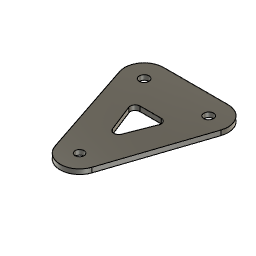
X Axis Support - Inside Support V2 (Autodesk Fusion 360 design; units mm, degrees)
Autodesk Fusion 360 part; units mm, degrees
sketch "Sketch1" plane through (0, 0, 0) normal (0, 0, 1) x (1, 0, 0) in component "X Axis Support - Inside Support V2"
  line L0 (0, 0) -> (64, 0)
  line L1 (64, 0) -> (64, 84)
  line L2 (64, 84) -> (0, 84)
  line L3 (0, 84) -> (0, 0)
  dimension "d1" = 64
  dimension "d2" = 84
  constraint horizontal L0
  constraint vertical L1
  constraint horizontal L2
  constraint vertical L3
  constraint coincident L0.start L3.end
  measures "d1" distance of L0.start L0.end
  measures "d2" distance of L0.start L2.end
extrude "Extrude1" add sketch "Sketch1" along normal blind 3 in component "X Axis Support - Inside Support V2"
sketch "Sketch2" plane through (0, 0, 3) normal (0, 0, 1) x (-1, 0, 0) in component "X Axis Support - Inside Support V2"
  line L0 (0, -84) -> (0, 0)
  line L1 (0, 0) -> (-64, 0)
  line L2 (-64, 0) -> (-64, -84)
  line L3 (-64, -84) -> (0, -84)
  line L4 (-12, -84) -> (-12, 0) construction
  line L5 (-52, -84) -> (-52, 0) construction
  line L6 (0, -12) -> (-64, -12) construction
  line L7 (0, -72) -> (-64, -72) construction
  circle A0 centre (-12, -72) radius 12
  circle A1 centre (-52, -72) radius 12
  circle A2 centre (-12, -72) radius 3
  circle A3 centre (-52, -72) radius 3
  line L8 (0, -72) -> (0, 0)
  line L9 (0, 0) -> (-32, 0)
  line L10 (-32, 0) -> (-64, 0)
  line L11 (-64, 0) -> (-64, -72)
  circle A4 centre (-32, -12) radius 12
  circle A5 centre (-32, -12) radius 2.75
  line L12 (0, -26) -> (-64, -26) construction
  line L13 (-12, 0) -> (0, -26)
  line L14 (-52, 0) -> (-64, -26)
  line L15 (0, -85) -> (-64, -85) construction
  line L16 (-32, -85) -> (-32, 0) construction
  line L17 (-0.6158, -68.2053) -> (-20.6158, -8.2053)
  line L18 (-63.3842, -68.2053) -> (-43.3842, -8.2053)
  line L19 (0, -56) -> (-64, -56) construction
  line L20 (0, -28) -> (-64, -28) construction
  line L21 (-21, -56) -> (-21, -28) construction
  line L22 (-43, -56) -> (-43, -28) construction
  line L23 (-21, -56) -> (-43, -56)
  line L24 (-32, -28) -> (-43, -56)
  line L25 (-32, -28) -> (-21, -56)
  dimension "d8" = 12
  dimension "d13" = 24
  dimension "d14" = 24
  dimension "d16" = 6
  dimension "d17" = 6
  dimension "d40" = 60
  dimension "d53" = 24
  dimension "d55" = 5.5
  dimension "d57" = 26
  dimension "d234" = 13
  dimension "d238" = 20
  dimension "d241" = 20
  dimension "d242" = 56
  dimension "d243" = 16
  dimension "d244" = 11
  dimension "d245" = 11
  constraint coincident L3 L4.start
  constraint coincident L1 L4.end
  constraint perpendicular L1 L4
  constraint coincident L3 L5.start
  constraint coincident L1 L5.end
  constraint perpendicular L1 L5
  constraint coincident L1 L9.end
  constraint coincident L0 L6.start
  constraint coincident L2 L6.end
  constraint perpendicular L2 L6
  constraint coincident L0 L7.start
  constraint coincident L2 L7.end
  constraint perpendicular L2 L7
  constraint coincident L7 A0.centre
  constraint coincident L4 A0.centre
  constraint coincident L7 A1.centre
  constraint coincident L5 A1.centre
  constraint concentric A0 A2
  constraint concentric A1 A3
  constraint coincident L0.end L1.start
  constraint coincident L1.end L2.start
  constraint coincident L6 A4.centre
  constraint concentric A4 A5
  constraint coincident L8 L12.start
  constraint coincident L11 L12.end
  constraint coincident L0 L15.start
  constraint coincident L2 L15.end
  constraint perpendicular L2 L15
  constraint midpoint L15 L16.start
  constraint perpendicular L9 L16
  constraint midpoint L6 A4.centre
  constraint tangent A0 L17
  constraint tangent A4 L17
  constraint coincident A4 L17.end
  constraint coincident A0 L17.start
  constraint coincident A4 L18.end
  constraint coincident A1 L18.start
  constraint tangent A1 L18
  constraint horizontal L19
  constraint coincident L8 L19.start
  constraint coincident L11 L19.end
  constraint coincident L8 L20.start
  constraint coincident L11 L20.end
  constraint coincident L19 L21.start
  constraint coincident L20 L21.end
  constraint perpendicular L20 L21
  constraint coincident L19 L22.start
  constraint coincident L20 L22.end
  constraint perpendicular L20 L22
  constraint midpoint L20 L24.start
  measures "d8" distance of L1 L6
  measures "d13" diameter of A0
  measures "d14" diameter of A1
  measures "d16" diameter of A2
  measures "d17" diameter of A3
  measures "d40" distance of L6 L7
  measures "d53" diameter of A4
  measures "d55" diameter of A5
  measures "d57" distance of L10 L12
  measures "d234" distance of A0.centre L15
  measures "d238" distance of L4 L16
  measures "d241" distance of L5 L16
  measures "d242" distance of L9 L19
  measures "d243" distance of L6 L20
  measures "d244" distance of L16 L21
  measures "d245" distance of L16 L22
extrude "Extrude2" cut sketch "Sketch2" against normal up to surface (3 mm away) contours L0 L3 A0 | L0 L1 A0 L8 L9 A4 L13 L17 | L0 L1 L8 L9 L13 | L2 L3 A1 | L1 L2 A1 L10 L11 A4 L14 L18 | L1 L2 L10 L11 L14 | A2 | A3 | A5 | L23 L24 L25 in component "X Axis Support - Inside Support V2"
fillet "Fillet11" radius 3 3 edges at (21, 56, 1.5) (43, 56, 1.5) (32, 28, 1.5) in component "X Axis Support - Inside Support V2"
component "X Axis Support - Inside Support V2" placed x (1, 0, 0) y (0, 1, 0) z (0, 0, 1) at (0, 0, 0)
named bodies: "X Axis Support - Inside Support V2"
